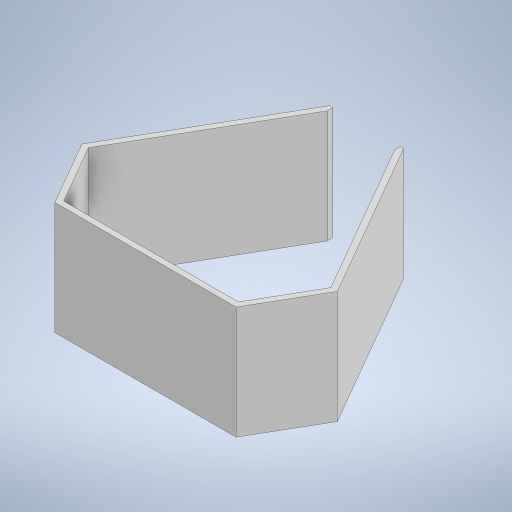
# Autodesk Inventor part: base_cover
Saved by Autodesk Inventor 2024.1 (Build 281209000, 209)
## iProperties
Created: 2025-03-10
Part Number: base_cover
Material: 一般
Document SubType Name: Modeling
Designer: hibik
Density: 1 g/cm^3
Appearance: 既定
Author: hibik
Autodesk Inventor part; units mm, degrees
ref_plane "YZ Plane" through (0, 0, 0) normal (1, 0, 0) x (0, 1, 0)
ref_plane "XZ Plane" through (0, 0, 0) normal (0, 1, 0) x (-1, 0, 0)
ref_plane "XY Plane" through (0, 0, 0) normal (0, 0, 1) x (1, 0, 0)
sketch "スケッチ1" plane through (0, 0, 0) normal (0, 1, 0) x (-1, 0, 0)
  line L0 (137.5, 79.3857) -> (-137.5, 79.3857)
  line L1 (-137.5, 79.3857) -> (0, -158.7713)
  line L2 (0, -158.7713) -> (137.5, 79.3857)
  line L3 (137.5, 79.3857) -> (-68.75, -39.6928) construction
  line L4 (77.5, 79.3857) -> (107.5, 27.4241)
  line L5 (-107.5, 27.4241) -> (-77.5, 79.3857)
  line L6 (30, -106.8098) -> (-30, -106.8098)
  line L7 (80.3868, 84.3857) -> (0, 84.3857)
  line L8 (80.3868, 84.3857) -> (96.8301, 55.9049)
  line L9 (0, 0) -> (0, 84.3857) construction
  line L10 (-80.3868, 84.3857) -> (0, 84.3857)
  line L11 (-80.3868, 84.3857) -> (-96.8301, 55.9049)
  line L12 (-113.2735, 27.4241) -> (-96.8301, 55.9049)
  line L13 (-113.2735, 27.4241) -> (-73.0801, -42.1928)
  line L14 (-32.8868, -111.8098) -> (-73.0801, -42.1928)
  line L15 (-32.8868, -111.8098) -> (0, -111.8098)
  line L16 (32.8868, -111.8098) -> (0, -111.8098)
  line L17 (32.8868, -111.8098) -> (73.0801, -42.1928)
  line L18 (113.2735, 27.4241) -> (73.0801, -42.1928)
  line L19 (113.2735, 27.4241) -> (96.8301, 55.9049)
  line L20 (30, -111.8098) -> (30, -106.8098)
  line L21 (-30, -111.8098) -> (-30, -106.8098)
  line L22 (-30, -106.8098) -> (30, -106.8098)
  point P0 (-30, -106.8098)
  point P1 (-107.5, 27.4241)
  point P2 (-77.5, 79.3857)
  point P3 (30, -106.8098)
  dimension "d0" = 275
  dimension "d1" = 60
  dimension "d4" = 360
  dimension "d6" = 5
  dimension "d7" = 5
  dimension "d10" = 360
  constraints: 46 end point, 9 point on line, 3 parallel, 3 perpendicular, 2 equal length, 2 symmetric about line, 2 vertical alignment, 1 horizontal, 1 midpoint, 1 vertical, 38 other
  measures "d0" distance of L0.start L0.end
  measures "d1" distance of L0.start L4.start
  measures "d6" distance between parallel lines of L7 L0
  measures "d7" distance between parallel lines of L4 L8
extrude "押し出し1" add sketch "スケッチ1" along normal blind 100 contours L0 L11 L10 L7 L8 | L0 L8 L19 L2 L4 | L5 L1 L12 L11 L0 | L2 L19 L18 L17 L16 L20 | L1 L21 L15 L14 L13 L12
